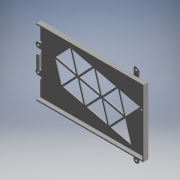
# Autodesk Inventor part: PCB_deck
Saved by Autodesk Inventor 2019 (Build 230136000, 136)
## iProperties
Part Number: PCB_deck
Material: Generic
Document SubType Name: Modeling
Designer: Jorge
Appearance: Default
Author: Jorge
Autodesk Inventor part; units mm, degrees
ref_plane "YZ Plane" through (0, 0, 0) normal (1, 0, 0) x (0, 1, 0)
ref_plane "XZ Plane" through (0, 0, 0) normal (0, 1, 0) x (-1, 0, 0)
ref_plane "XY Plane" through (0, 0, 0) normal (0, 0, 1) x (1, 0, 0)
sketch "Sketch1" plane through (0, 0, 0) normal (0, 0, 1) x (1, 0, 0)
  line L0 (151.1, 1.6) -> (0, 1.6)
  line L1 (1.6, 24.1) -> (1.6, 71.6)
  line L2 (1.6, 24.1) -> (0, 24.1)
  line L3 (1.6, 47.85) -> (151.1, 47.85) construction
  line L4 (1.6, 71.6) -> (0, 71.6)
  line L5 (0, 71.6) -> (0, 94.1)
  line L6 (1.6, 30.975) -> (-2.9, 30.975) construction
  circle A0 centre (-2.9, 30.975) radius 1.5
  line L7 (-2.9, 27.225) -> (-2.9, 34.725) construction
  line L8 (-2.9, 27.225) -> (1.6, 27.225)
  line L9 (-2.9, 34.725) -> (1.6, 34.725)
  line L10 (1.6, 57.85) -> (0, 57.85)
  line L11 (0, 57.85) -> (0, 37.85)
  line L12 (0, 37.85) -> (1.6, 37.85)
  line L13 (0, 57.85) -> (0, 68.475) construction
  line L14 (0, 37.85) -> (0, 27.225) construction
  line L15 (0, 24.1) -> (0, 34.725) construction
  line L16 (152.7, 0) -> (0, 0)
  line L17 (152.7, 95.7) -> (0, 95.7)
  line L18 (0, 95.7) -> (0, 94.1)
  line L19 (0, 94.1) -> (151.1, 94.1)
  line L20 (137.1, 94.1) -> (137.1, 103.95) construction
  circle A1 centre (137.1, 103.95) radius 1.5
  arc A2 (140.85, 103.95) -> (133.35, 103.95) centre (137.1, 103.95) ccw
  line L21 (133.35, 103.95) -> (140.85, 103.95) construction
  line L22 (140.85, 103.95) -> (140.85, 95.7)
  line L23 (133.35, 103.95) -> (133.35, 95.7)
  line L24 (137.1, 1.6) -> (137.1, -8.25) construction
  circle A3 centre (137.1, -8.25) radius 1.5
  arc A4 (133.35, -8.25) -> (140.85, -8.25) centre (137.1, -8.25) ccw
  line L25 (133.35, -8.25) -> (140.85, -8.25) construction
  line L26 (140.85, -8.25) -> (140.85, 0)
  line L27 (133.35, -8.25) -> (133.35, 0)
  arc A5 (-2.9, 34.725) -> (-2.9, 27.225) centre (-2.9, 30.975) ccw
  line L28 (151.1, 94.1) -> (151.1, 1.6)
  line L29 (152.7, 0) -> (152.7, 95.7)
  line L30 (0, 24.1) -> (0, 0)
  line L31 (1.6, 64.725) -> (-2.9, 64.725) construction
  circle A6 centre (-2.9, 64.725) radius 1.5
  line L32 (-2.9, 68.475) -> (-2.9, 60.975) construction
  line L33 (1.6, 68.475) -> (-2.9, 68.475)
  line L34 (1.6, 60.975) -> (-2.9, 60.975)
  arc A7 (-2.9, 68.475) -> (-2.9, 60.975) centre (-2.9, 64.725) ccw
  point P0 (0, 0)
  dimension "d8" = 3
  dimension "d9" = 4.5
  dimension "d11" = 1.6
  dimension "d14" = 3
  dimension "d15" = 7.5
  dimension "d17" = 7.5
  dimension "d19" = 112.2
  dimension "d23" = 1.6
  dimension "d27" = 22.5
  dimension "d28" = 1.6
  dimension "d29" = 1.6
  dimension "d30" = 149.5
  dimension "d31" = 92.5
  dimension "d32" = 1.6
  dimension "d34" = 140
  dimension "d36" = 33.75
  dimension "d37" = 7.5
  constraints: 68 end point, 16 symmetric about line, 10 point on line, 9 vertical, 8 centre point, 8 point on circle, 6 horizontal, 6 perpendicular, 5 coincident, 5 midpoint, 4 tangent, 3 equal length, 3 parallel, 17 other
  measures "d8" diameter of A0
  measures "d9" distance of L7.start L8.end
  measures "d11" distance of L12.end L11.end
  measures "d14" diameter of A1
  measures "d15" distance between parallel lines of L9 L8
  measures "d17" distance between parallel lines of L22 L23
  measures "d19" distance between parallel lines of L25 L21
  measures "d23" distance between parallel lines of L17 L19
  measures "d27" distance between parallel lines of L0 L2
  measures "d28" distance between parallel lines of L28 L29
  measures "d29" distance between parallel lines of L0 L16
  measures "d31" distance between parallel lines of L19 L0
  measures "d32" distance of L2.start L2.end
  measures "d34" distance between parallel lines of L24 L7
  measures "d36" distance between parallel lines of L6 L31
  measures "d37" distance between parallel lines of L33 L34
extrude "Extrusion1" add sketch "Sketch1" along normal blind 1.6
extrude "Extrusion2" add sketch "Sketch1" along normal blind 7 contours L28 L19 L18 L17 L29 L16 L30 L0 | L12 L11 L10 L1
sketch "Sketch2" plane through (151.1, 1.6, 1.6) normal (-1, 0, 0) x (0, 0, 1)
  line L0 (-1.6, -1.6) -> (-1.6, 94.1) projected
  line L1 (-1.6, 94.1) -> (5.4, 94.1) projected
  line L2 (5.4, -1.6) -> (5.4, 94.1) projected
  line L3 (-1.6, -1.6) -> (5.4, -1.6) projected
  line L4 (0, 56.25) -> (0, 36.25) projected
  line L5 (0, 36.25) -> (0, 33.125) projected
  line L6 (0, 33.125) -> (0, 25.625) projected
  line L7 (0, 25.625) -> (0, 22.5) projected
  line L8 (0, 22.5) -> (0, 0) projected
  line L9 (0, 0) -> (0, 92.5) projected
  line L10 (0, 92.5) -> (0, 70) projected
  line L11 (0, 70) -> (0, 66.875) projected
  line L12 (0, 66.875) -> (0, 59.375) projected
  line L13 (0, 59.375) -> (0, 56.25) projected
  line L14 (0, 64.625) -> (0, 61.625) projected
  line L15 (0, 30.875) -> (0, 27.875) projected
  line L16 (5.4, -1.6) -> (5.4, 94.1) projected
  line L17 (5.4, 61.25) -> (3.4, 61.25)
  line L18 (3.4, 61.25) -> (3.4, 31.25)
  line L19 (3.4, 31.25) -> (5.4, 31.25)
  line L20 (5.4, 31.25) -> (5.4, 61.25)
  line L21 (-1.6, -1.6) -> (-1.6, 94.1) projected
  line L22 (5.4, 46.25) -> (-1.6, 46.25) construction
  dimension "d42" = 2
  dimension "d43" = 30
  constraints: 10 end point, 2 midpoint, 2 parallel, 1 horizontal, 1 perpendicular, 1 point on line, 1 other
  measures "d42" distance of L19.end L18.end
  measures "d43" distance between parallel lines of L19 L17
extrude "Extrusion3" add sketch "Sketch2" along normal blind 3.5 contours L19 L18 L17 L2
chamfer "Chamfer1" distance 2 angle 45 1 edges at (147.6, 47.85, 5)
sketch "Sketch3" plane through (1.6, 37.85, 1.6) normal (1, 0, 0) x (0, 0, -1)
  line L0 (1.6, 20) -> (1.6, 0) projected
  line L1 (1.6, 0) -> (-5.4, 0) projected
  line L2 (-5.4, 20) -> (-5.4, 0) projected
  line L3 (1.6, 20) -> (-5.4, 20) projected
  line L4 (1.6, 0) -> (-5.4, 0) projected
  line L5 (1.6, 20) -> (-5.4, 20) projected
  line L6 (-5.4, 0) -> (-3.2, 0)
  line L7 (-3.2, 0) -> (-3.2, 20)
  line L8 (-3.2, 20) -> (-5.4, 20)
  line L9 (-5.4, 20) -> (-5.4, 0)
  point P0 (1.6, -37.85)
  dimension "d49" = 2.2
  constraints: 8 end point, 2 parallel, 1 horizontal, 1 perpendicular, 1 point on line
  measures "d49" distance of L8.end L7.end
extrude "Extrusion4" add sketch "Sketch3" along normal blind 2 contours L7 L1 L2 L3
chamfer "Chamfer2" distance 0.75 angle 45 2 edges at (3.6, 47.85, 7) (3.6, 47.85, 4.8)
sketch "Sketch4" plane through (0, 0, 0) normal (0, 0, 1) x (1, 0, 0)
  line L0 (22.2208, 62.4088) -> (42.8238, 84.2151)
  line L1 (42.8238, 84.2151) -> (51.4072, 55.4693)
  line L2 (51.4072, 55.4693) -> (22.2208, 62.4088)
  line L3 (14.9452, 64.1387) -> (113.2518, 40.7647) construction
  line L4 (56.2716, 54.3127) -> (76.8746, 76.1191)
  line L5 (76.8746, 76.1191) -> (85.4579, 47.3732)
  line L6 (85.4579, 47.3732) -> (56.2716, 54.3127)
  line L7 (74.4424, 76.6973) -> (53.8394, 54.891)
  line L8 (53.8394, 54.891) -> (45.256, 83.6369)
  line L9 (45.256, 83.6369) -> (74.4424, 76.6973)
  line L10 (97.3632, 71.2476) -> (-0.9434, 94.6215) construction
  line L11 (131.414, 63.1515) -> (33.1073, 86.5254) construction
  line L12 (87.8901, 46.7949) -> (79.3067, 75.5408)
  line L13 (79.3067, 75.5408) -> (108.4931, 68.6013)
  line L14 (108.4931, 68.6013) -> (87.8901, 46.7949)
  line L15 (165.4647, 55.0554) -> (67.158, 78.4293) construction
  line L16 (121.9409, 38.6988) -> (113.3575, 67.4447)
  line L17 (113.3575, 67.4447) -> (142.5438, 60.5052)
  line L18 (142.5438, 60.5052) -> (121.9409, 38.6988)
  line L19 (90.3223, 46.2166) -> (110.9253, 68.023)
  line L20 (110.9253, 68.023) -> (119.5087, 39.2771)
  line L21 (119.5087, 39.2771) -> (90.3223, 46.2166)
  line L22 (130.3709, 35.4096) -> (6.002, 64.9802) construction
  line L23 (21.6425, 59.9766) -> (30.2259, 31.2307)
  line L24 (30.2259, 31.2307) -> (50.8289, 53.0371)
  line L25 (50.8289, 53.0371) -> (21.6425, 59.9766)
  line L26 (55.6933, 51.8805) -> (64.2767, 23.1346)
  line L27 (64.2767, 23.1346) -> (84.8796, 44.941)
  line L28 (84.8796, 44.941) -> (55.6933, 51.8805)
  line L29 (61.8445, 23.7129) -> (53.2611, 52.4588)
  line L30 (53.2611, 52.4588) -> (32.6581, 30.6524)
  line L31 (32.6581, 30.6524) -> (61.8445, 23.7129)
  line L32 (118.8161, 10.167) -> (20.5094, 33.541) construction
  line L33 (87.3118, 44.3627) -> (66.7089, 22.5563)
  line L34 (66.7089, 22.5563) -> (95.8952, 15.6168)
  line L35 (95.8952, 15.6168) -> (87.3118, 44.3627)
  line L36 (121.3626, 36.2666) -> (100.7596, 14.4602)
  line L37 (100.7596, 14.4602) -> (129.946, 7.5207)
  line L38 (129.946, 7.5207) -> (121.3626, 36.2666)
  line L39 (89.744, 43.7844) -> (98.3274, 15.0385)
  line L40 (98.3274, 15.0385) -> (118.9304, 36.8449)
  line L41 (118.9304, 36.8449) -> (89.744, 43.7844)
  dimension "d59" = 35
  dimension "d76" = 2.5
  dimension "d77" = 30
  dimension "d80" = 35
  dimension "d85" = 1.25
  constraints: 84 end point, 20 symmetric about line, 6 equal length, 3 collinear, 2 parallel, 1 point on line, 31 other
  measures "d59" distance of L0.start L4.start
  measures "d76" distance of L1.end L7.end
  measures "d77" distance of L0.start L0.end
  measures "d80" distance of L10.start L11.start
  measures "d85" distance between parallel lines of L22 L3
extrude "Extrusion5" cut sketch "Sketch4" along normal through all
equation "\"dis\" = 5"
equation "\"d73\" = 5"
body "Solid1"
